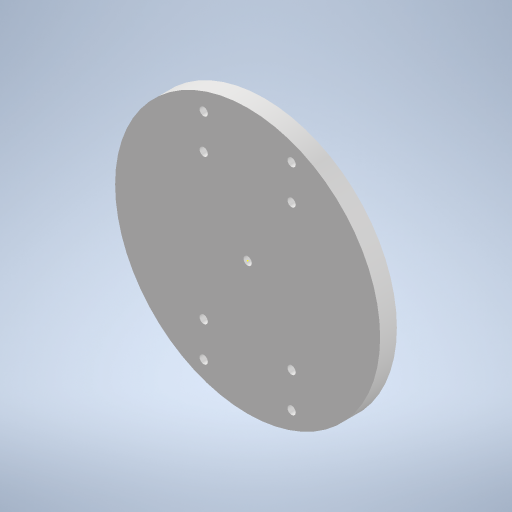
# Autodesk Inventor part: podstawa
Saved by Autodesk Inventor 2023 (Build 270158000, 158)
## iProperties
Created: 2022-11-02
Part Number: podstawa
Material: Generic
Document SubType Name: Modeling
Designer: Kamil
Density: 1 g/cm^3
Appearance: Default
Author: Kamil
Autodesk Inventor part; units mm, degrees
ref_plane "YZ Plane" through (0, 0, 0) normal (1, 0, 0) x (0, 1, 0)
ref_plane "XZ Plane" through (0, 0, 0) normal (0, 1, 0) x (-1, 0, 0)
ref_plane "XY Plane" through (0, 0, 0) normal (0, 0, 1) x (1, 0, 0)
sketch "Sketch1" plane through (0, 0, 0) normal (0, 0, 1) x (1, 0, 0)
  circle A0 centre (0, 0) radius 47.5
  dimension "d0" = 95
  constraints: 1 centre point, 1 coincident
  measures "d0" diameter of A0
extrude "Extrusion1" add sketch "Sketch1" along normal blind 6
sketch "Sketch12" plane through (0, 0, 0) normal (0, 0, -1) x (-1, 0, 0)
  line L0 (15.75, 36.5709) -> (15.75, -44.8128)
  circle A0 centre (0, 0) radius 47.5 projected
  line L1 (-15.75, 36.5709) -> (-15.75, -44.8128)
  line L2 (-15.75, 36.5709) -> (-15.75, 44.8128)
  line L3 (15.75, 36.5709) -> (15.75, 45.8997)
  line L4 (0, 0) -> (0, 26)
  line L5 (0, 26) -> (0, -26)
  line L6 (0, -26) -> (15.75, -26)
  line L7 (-15.75, -26) -> (0, -26)
  line L8 (0, 26) -> (15.75, 26)
  line L9 (-15.75, 26) -> (0, 26)
  circle A1 centre (-15.75, 26) radius 1.5
  circle A2 centre (15.75, 26) radius 1.5
  circle A3 centre (15.75, -26) radius 1.5
  circle A4 centre (-15.75, -26) radius 1.5
  line L10 (-15.75, 26) -> (-15.75, 38.5)
  line L11 (-15.75, 38.5) -> (15.75, 38.5)
  circle A5 centre (-15.75, 38.5) radius 1.5
  circle A6 centre (15.75, 38.5) radius 1.5
  line L12 (-15.75, -26) -> (-15.75, -38.5)
  line L13 (-15.75, -38.5) -> (15.75, -38.5)
  circle A7 centre (15.75, -38.5) radius 1.5
  circle A8 centre (-15.75, -38.5) radius 1.5
  constraints: 28 end point, 12 point on line, 8 centre point, 8 coincident, 4 perpendicular, 3 point on circle, 2 collinear, 1 parallel, 1 vertical
extrude "Extrusion2" cut sketch "Sketch12" against normal blind 10 contours A2 L0 | L0 L8 A2 | A6 L11 L3 | L3 A6 | L0 A2 L8 | L11 A6 L3 | A5 L2 L11 | L11 L2 A5 | A3 L0 | L0 L6 A3 | A1 L1 L9 | L9 L1 A1 | L2 A5 | L0 A3 L6 | L1 A1 | A4 L1 L7 | L7 L1 A4 | L1 A4 | A7 L0 | L0 L13 A7 | A7 L13 L0 | A8 L1 | L1 L13 A8 | A8 L13 L1
sketch "Sketch14" plane through (0, 0, 6) normal (0, 0, 1) x (1, 0, 0)
  point P0 (0, 0)
sketch "Sketch15" plane through (0, 0, 6) normal (0, 0, 1) x (1, 0, 0)
  circle A0 centre (0, 0) radius 1.5
  dimension "d22" = 3
  constraints: 1 centre point, 1 coincident
  measures "d22" diameter of A0
extrude "Extrusion4" cut sketch "Sketch15" against normal blind 10
body "Solid1"
